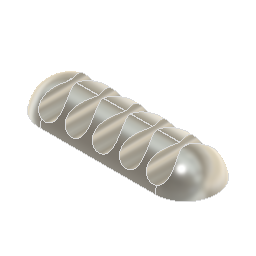
Круглое пятиярдное крепление проводов (Autodesk Fusion 360 design; units mm, degrees)
Autodesk Fusion 360 part; units mm, degrees
sketch "Sketch1" plane through (0, 0, 0) normal (0, 0, 1) x (1, 0, 0)
  line L0 (-17, -9) -> (17, -9)
  arc A0 (17, -9) -> (17, 9) centre (17, 0) ccw
  line L1 (17, 9) -> (-17, 9)
  arc A1 (-17, 9) -> (-17, -9) centre (-17, 0) ccw
  line L2 (-17, 0) -> (17, 0) construction
  dimension "d1" = 18
  constraint tangent L0 A0
  constraint tangent A0 L1
  constraint parallel L0 L1
  constraint tangent L1 A1
  constraint tangent L0 A1
  constraint horizontal L2
  constraint midpoint L2 origin
  measures "d1" diameter of A0
extrude "Extrude1" add sketch "Sketch1" along normal blind 8
fillet "Fillet1" radius 9 4 edges at (26, 0, 8) (0, 9, 8) (-26, 0, 8) (0, -9, 8)
sketch "Sketch2" plane through (0, 0, 0) normal (0, 1, 0) x (1, 0, 0)
  circle A0 centre (0, -5) radius 3.1
  circle A1 centre (8, -5) radius 3.1
  circle A2 centre (16, -5) radius 3.1
  circle A3 centre (-8, -5) radius 3.1
  circle A4 centre (-16, -5) radius 3.1
  circle A5 centre (0, -5) radius 3.1
  dimension "d6" = 6.2
  dimension "d7" = 6.2
  dimension "d8" = 6.2
  dimension "d9" = 6.2
  dimension "d10" = 6.2
  dimension "d11" = 6.2
  measures "d6" diameter of A0
  measures "d7" diameter of A1
  measures "d8" diameter of A2
  measures "d9" diameter of A3
  measures "d10" diameter of A4
  measures "d11" diameter of A5
extrude "Extrude2" cut sketch "Sketch2" along normal mid plane 40
